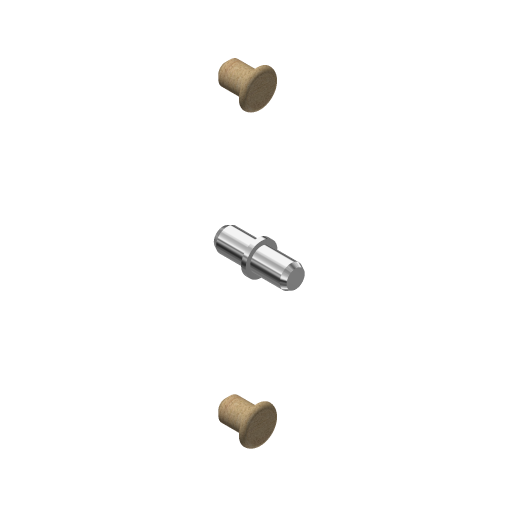
# Autodesk Inventor part: Shelf support D5 L16
Saved by Autodesk Inventor 2024 (Build 280153000, 153)
## iProperties
Category: Holders
Created: 2013-11-08
Part Number: Shelf support D5 L16
Material: Generic
Document SubType Name: Modeling
Designer: G. K.
Authority: Design by UAB Čeli APS
Density: 1 g/cm^3
Appearance: Default
Description: Shelf holder
Mase: 0.0
Author: G. K.
Title: Shelf holder
Subject: Shelf hangers
Keywords: Shelf hanger, holder, D5, L16
Comments: Shelf hanger, holder, D5, L16, Shelf holder
Revision Number: 1
Autodesk Inventor part; units mm, degrees
ref_plane "YZ Plane" through (0, 0, 0) normal (1, 0, 0) x (0, 1, 0)
ref_plane "XZ Plane" through (0, 0, 0) normal (0, 1, 0) x (-1, 0, 0)
ref_plane "XY Plane" through (0, 0, 0) normal (0, 0, 1) x (1, 0, 0)
sketch "Sketch2" plane through (0, 0, 0) normal (0, 1, 0) x (-1, 0, 0)
  line L0 (13, 0) -> (13, -2.5)
  line L1 (13, -2.5) -> (-13, -2.5)
  line L2 (-13, -2.5) -> (-13, 0)
  line L3 (-13, 0) -> (13, 0)
  line L4 (13, 0) -> (14.4434, 0)
  line L5 (14.4434, 0) -> (13, -2.5)
  line L6 (-13, 0) -> (-14.4434, 0)
  point P0 (0, 0)
  point P1 (0, 0)
  point P2 (0, 0)
  dimension "d0" = 60
  dimension "d1" = 5
  dimension "d2" = 13
  constraints: 14 end point, 3 collinear, 2 parallel, 1 coincident, 1 midpoint, 1 perpendicular
  measures "d0" angle of L5 L4
  measures "d1" diameter of L1 L3
  measures "d2" distance from line of point (0, 0) L0
revolve "Revolution1" add sketch "Sketch2" angle 360 about axis through (13, 0, 0) along (-1, 0, 0)
sketch "Sketch3" plane through (0, 0, 0) normal (0, 1, 0) x (-1, 0, 0)
  line L0 (-8, 0) -> (8, 0)
  line L1 (8, 0) -> (8, 2)
  line L2 (8, 2) -> (7, 2.5)
  line L3 (7, 2.5) -> (0.5, 2.5)
  line L4 (0.5, 2.5) -> (0.5, 3.5)
  line L5 (0.5, 3.5) -> (-0.5, 3.5)
  line L6 (-0.5, 3.5) -> (-0.5, 2.5)
  line L7 (-0.5, 2.5) -> (-7, 2.5)
  line L8 (-7, 2.5) -> (-8, 2)
  line L9 (-8, 2) -> (-8, 0)
  line L10 (0, 0) -> (0, 3.5) construction
  dimension "d4" = 16
  dimension "d5" = 1
  dimension "d6" = 7
  dimension "d7" = 5
  dimension "d8" = 1
  dimension "d9" = 4
  constraints: 23 end point, 4 parallel, 2 midpoint, 2 perpendicular, 1 coincident, 1 collinear, 1 horizontal, 1 symmetric about line, 1 vertical, 1 other
  measures "d4" distance of L0.start L0.end
  measures "d5" distance between parallel lines of L4 L6
  measures "d6" diameter of L5 L0
  measures "d7" diameter of L7 L0
  measures "d8" horizontal distance of L7.end L8.end
  measures "d9" diameter of L8.end L0
revolve "Revolution2" add sketch "Sketch3" angle 360 about axis through (8, 0, 0) along (-1, 0, 0) separate body
pattern_linear "Rectangular Pattern1" count 3 spacing 32 along (0, 0, 1) first direction both ways yes bodies 1
sketch "Sketch4" plane through (0, 0, 0) normal (0, 1, 0) x (-1, 0, 0)
  line L0 (19.0516, 32) -> (-26.6641, 32)
  line L1 (6.5, 34.5) -> (0.5, 34.5)
  line L2 (0.5, 34.5) -> (0.5, 36)
  line L3 (0.5, 36) -> (0.5, 36)
  line L4 (-0.5, 35) -> (-0.5, 32)
  line L5 (7.5, 33.5) -> (7.5, 32)
  line L6 (6.5, 34.5) -> (7.5, 33.5)
  arc A0 (0.5, 36) -> (-0.5, 35) centre (0.5, 35) ccw
  point P0 (0, 0)
  point P1 (7.5, 34.5)
  dimension "d14" = 32
  dimension "d15" = 7
  dimension "d16" = 5
  dimension "d17" = 8
  dimension "d18" = 1
  dimension "d20" = 1
  dimension "d21" = 1
  dimension "d22" = 1
  dimension "d23" = 0.5
  constraints: 14 end point, 4 point on line, 3 perpendicular, 2 parallel, 2 point on circle, 2 tangent, 1 centre point, 1 horizontal
  measures "d14" distance from line of L0 point (0, 0)
  measures "d15" distance of point (7.5, 34.5) L1.end
  measures "d16" diameter of L1 L0
  measures "d17" diameter of L3 L0
  measures "d18" distance between parallel lines of L2 L4
  measures "d20" distance of L1.start point (7.5, 34.5)
  measures "d21" distance of L5.start point (7.5, 34.5)
  measures "d22" radius of A0
  measures "d23" distance from line of L2 point (0, 0)
revolve "Up Cap" add sketch "Sketch4" angle 360 about axis through (-19.0516, 0, 32) along (1, 0, 0) separate body
sketch "Sketch5" plane through (0, 0, 0) normal (0, 1, 0) x (-1, 0, 0)
  line L0 (17.6496, -32) -> (-28.0661, -32)
  line L1 (6.5, -29.5) -> (0.5, -29.5)
  line L2 (0.5, -29.5) -> (0.5, -28)
  line L3 (-0.5, -29) -> (-0.5, -32)
  line L4 (7.5, -30.5) -> (7.5, -32)
  line L5 (6.5, -29.5) -> (7.5, -30.5)
  arc A0 (0.5, -28) -> (-0.5, -29) centre (0.5, -29) ccw
  line L6 (0.5, 28) -> (0.5, 36) projected
  point P0 (0, 0)
  point P1 (0, -11.9071)
  point P2 (7.5, -29.5)
  dimension "d32" = 7
  dimension "d33" = 5
  dimension "d34" = 8
  dimension "d35" = 1
  dimension "d36" = 1
  dimension "d37" = 1
  dimension "d38" = 1
  dimension "d39" = 0.5
  dimension "d40" = 32
  constraints: 12 end point, 4 point on line, 3 perpendicular, 2 horizontal, 2 point on circle, 1 centre point, 1 coincident, 1 parallel, 1 tangent, 3 other
  measures "d32" distance of point (7.5, -29.5) L1.end
  measures "d33" diameter of L1 L0
  measures "d35" distance between parallel lines of L2 L3
  measures "d36" distance of L1.start point (7.5, -29.5)
  measures "d37" distance of L4.start point (7.5, -29.5)
  measures "d38" radius of A0
  measures "d39" distance from line of L2 point (0, -11.907)
  measures "d40" vertical distance of point (0, 0) L0.end
revolve "Down Cap" add sketch "Sketch5" angle 360 about axis through (-17.6496, 0, -32) along (1, 0, 0) separate body
pattern_linear "Up Pattern" [suppressed]
pattern_linear "Down Pattern" [suppressed]
equation "\"d21\" = d20"
equation "\"d37\" = d36"
